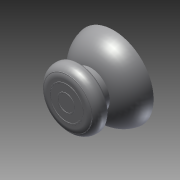
# Autodesk Inventor part: Control Stick
Saved by Autodesk Inventor 2012 SP1 (Build 160190100, 190)
## iProperties
Created: 2011-12-20
Part Number: Control Stick
Material: Default
Document SubType Name: Modeling
Designer: 133098
Density: 1 g/cm^3
Author: 133098
Autodesk Inventor part; units mm, degrees
ref_plane "YZ Plane" through (0, 0, 0) normal (1, 0, 0) x (0, 1, 0)
ref_plane "XZ Plane" through (0, 0, 0) normal (0, 1, 0) x (-1, 0, 0)
ref_plane "XY Plane" through (0, 0, 0) normal (0, 0, 1) x (1, 0, 0)
sketch "Sketch1" plane through (0, 0, 0) normal (0, 0, 1) x (1, 0, 0)
  circle A0 centre (0, 0) radius 10.795
  dimension "d0" = 21.59
  constraints: 1 centre point, 1 coincident
  measures "d0" diameter of A0
extrude "Extrusion1" add sketch "Sketch1" along normal blind 6.35
fillet "Fillet1" radius 7.62 1 edges at (-10.795, 0, 6.35)
sketch "Sketch2" plane through (0, 0, 0) normal (0, 0, -1) x (-1, 0, 0)
  circle A0 centre (0, 0) radius 10.795 projected
  circle A1 centre (0, 0) radius 5.08
  dimension "d4" = 10.16
  constraints: 1 centre point, 1 coincident
  measures "d4" diameter of A1
extrude "Extrusion2" add sketch "Sketch2" against normal blind 9.144 contours A1
sketch "Sketch3" plane through (0, 0, 9.144) normal (0, 0, 1) x (1, 0, 0)
  circle A0 centre (0, 0) radius 5.08 projected
  circle A1 centre (0, 0) radius 7.874
  dimension "d7" = 15.748
  constraints: 1 centre point, 1 coincident
  measures "d7" diameter of A1
extrude "Extrusion3" add sketch "Sketch3" along normal blind 3.556 contours A0 | A1
fillet "Fillet2" radius 2.54 1 edges at (-7.874, 0, 12.7)
fillet "Fillet3" radius 0.635 1 edges at (-7.874, 0, 9.144)
sketch "Sketch4" plane through (0, 0, 9.144) normal (0, 0, -1) x (-1, 0, 0)
  circle A0 centre (0, 0) radius 5.08 projected
  circle A1 centre (0, 0) radius 7.239 projected
  circle A2 centre (0, 0) radius 6.604
  circle A3 centre (0, 0) radius 5.969
  dimension "d12" = 13.208
  dimension "d13" = 11.938
  constraints: 3 coincident, 2 centre point
  measures "d12" diameter of A2
  measures "d13" diameter of A3
extrude "Extrusion4" add sketch "Sketch4" against normal blind 3.302 contours A2
fillet "Fillet4" radius 0.0635 1 edges at (6.604, 0, 12.446)
sketch "Sketch5" plane through (0, 0, 9.144) normal (0, 0, -1) x (-1, 0, 0)
  circle A0 centre (0, 0) radius 7.239 projected
  circle A1 centre (0, 0) radius 5.08 projected
  circle A2 centre (0, 0) radius 4.572
  circle A3 centre (0.1199, 0) radius 4.191
  dimension "d17" = 9.144
  dimension "d18" = 8.382
  constraints: 2 centre point, 2 coincident
  measures "d17" diameter of A2
  measures "d18" diameter of A3
extrude "Extrusion5" add sketch "Sketch5" against normal blind 3.6195 contours A2
fillet "Fillet5" radius 0.0635 2 edges at (4.0711, 0, 12.7635) (4.572, 0, 12.7635)
sketch "Sketch6" plane through (-0.1199, 0, 12.7) normal (0, 0, 1) x (1, 0, 0)
  circle A0 centre (0, 0) radius 4.191 projected
  circle A1 centre (0, 0) radius 2.413
  circle A2 centre (0, 0) radius 2.032
  point P0 (0.1199, 0)
  dimension "d22" = 4.826
  dimension "d23" = 4.064
  constraints: 2 centre point, 2 coincident
  measures "d22" diameter of A1
  measures "d23" diameter of A2
extrude "Extrusion6" add sketch "Sketch6" along normal blind 0.0635 contours A1
fillet "Fillet6" radius 0.0635 2 edges at (-2.1519, 0, 12.7635) (-2.5329, 0, 12.7635)
body "Solid1"
